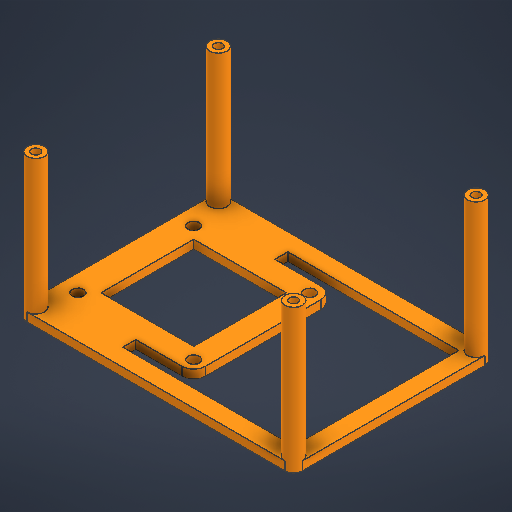
# Autodesk Inventor part: fan_support
Saved by Autodesk Inventor 2026.1 (Build 301233000, 233)
## iProperties
Created: 2026-04-26
Part Number: fan_support
Material: Generic
Document SubType Name: Modeling
Designer: emanuel
Density: 1 g/cm^3
Appearance: Default
Author: emanuel
Autodesk Inventor part; units mm, degrees
ref_plane "YZ Plane" through (0, 0, 0) normal (1, 0, 0) x (0, 1, 0)
ref_plane "XZ Plane" through (0, 0, 0) normal (0, 1, 0) x (-1, 0, 0)
ref_plane "XY Plane" through (0, 0, 0) normal (0, 0, 1) x (1, 0, 0)
sketch "Sketch1" plane through (0, 0, 0) normal (0, 1, 0) x (-1, 0, 0)
  line L0 (0, 0) -> (40, 0)
  line L1 (40, 0) -> (40, -40)
  line L2 (40, -40) -> (0, -40)
  line L3 (0, -40) -> (0, 0)
  circle A0 centre (40, 0) radius 2
  circle A1 centre (40, -40) radius 2
  circle A2 centre (0, -40) radius 2
  circle A3 centre (0, 0) radius 2
  line L4 (40, -20) -> (43, -20)
  line L5 (43, 11.5) -> (43, -51.5)
  circle A4 centre (43, 11.5) radius 1.5
  circle A5 centre (43, -51.5) radius 1.5
  line L6 (43, 11.5) -> (-46, 11.5)
  line L7 (-46, 11.5) -> (-46, -51.5)
  line L8 (-46, -51.5) -> (43, -51.5)
  line L9 (43, -51.5) -> (43, 11.5)
  circle A6 centre (-46, 11.5) radius 1.5
  circle A7 centre (-46, -51.5) radius 1.5
  line L10 (-46, 11.5) -> (-46, -51.5) construction
  line L11 (-49, 11.5) -> (-49, -51.5)
  line L12 (-43, -51.5) -> (-43, 11.5)
  arc A8 (-43, 11.5) -> (-49, 11.5) centre (-46, 11.5) ccw
  arc A9 (-49, -51.5) -> (-43, -51.5) centre (-46, -51.5) ccw
  line L13 (-46, 11.5) -> (43, 11.5) construction
  line L14 (-46, 8.5) -> (43, 8.5)
  line L15 (43, 14.5) -> (-46, 14.5)
  arc A10 (-46, 14.5) -> (-46, 8.5) centre (-46, 11.5) ccw
  arc A11 (43, 8.5) -> (43, 14.5) centre (43, 11.5) ccw
  line L16 (43, 11.5) -> (43, -51.5) construction
  line L17 (40, 11.5) -> (40, -51.5)
  line L18 (46, -51.5) -> (46, 11.5)
  arc A12 (46, 11.5) -> (40, 11.5) centre (43, 11.5) ccw
  arc A13 (40, -51.5) -> (46, -51.5) centre (43, -51.5) ccw
  line L19 (43, -51.5) -> (-46, -51.5) construction
  line L20 (43, -48.5) -> (-46, -48.5)
  line L21 (-46, -54.5) -> (43, -54.5)
  arc A14 (43, -54.5) -> (43, -48.5) centre (43, -51.5) ccw
  arc A15 (-46, -48.5) -> (-46, -54.5) centre (-46, -51.5) ccw
  line L22 (40, 0) -> (0, 0) construction
  line L23 (40, 4) -> (0, 4)
  line L24 (0, -4) -> (40, -4)
  arc A16 (40, -4) -> (40, 4) centre (40, 0) ccw
  arc A17 (0, 4) -> (0, -4) centre (0, 0) ccw
  line L25 (40, 0) -> (40, -40) construction
  line L26 (36, 0) -> (36, -40)
  line L27 (44, -40) -> (44, 0)
  arc A18 (44, 0) -> (36, 0) centre (40, 0) ccw
  arc A19 (36, -40) -> (44, -40) centre (40, -40) ccw
  line L28 (40, -40) -> (0, -40) construction
  line L29 (40, -36) -> (0, -36)
  line L30 (0, -44) -> (40, -44)
  arc A20 (40, -44) -> (40, -36) centre (40, -40) ccw
  arc A21 (0, -36) -> (0, -44) centre (0, -40) ccw
  line L31 (0, -40) -> (0, 0) construction
  line L32 (4, -40) -> (4, 0)
  line L33 (-4, 0) -> (-4, -40)
  arc A22 (-4, -40) -> (4, -40) centre (0, -40) ccw
  arc A23 (4, 0) -> (-4, 0) centre (0, 0) ccw
  line L34 (20, 0) -> (20, 11.5) construction
  line L35 (24, 0) -> (24, 11.5)
  line L36 (16, 11.5) -> (16, 0)
  arc A24 (16, 0) -> (24, 0) centre (20, 0) ccw
  arc A25 (24, 11.5) -> (16, 11.5) centre (20, 11.5) ccw
  line L37 (20, -40) -> (20, -51.5) construction
  line L38 (16, -40) -> (16, -51.5)
  line L39 (24, -51.5) -> (24, -40)
  arc A26 (24, -40) -> (16, -40) centre (20, -40) ccw
  arc A27 (16, -51.5) -> (24, -51.5) centre (20, -51.5) ccw
  line L40 (40, -20) -> (43, -20) construction
  line L41 (40, -24) -> (43, -24)
  line L42 (43, -16) -> (40, -16)
  arc A28 (40, -16) -> (40, -24) centre (40, -20) ccw
  arc A29 (43, -24) -> (43, -16) centre (43, -20) ccw
  point P0 (-46, -20)
  point P1 (-1.5, 11.5)
  point P2 (-1.5, -51.5)
  point P3 (0, -20)
  point P4 (20, 5.75)
  point P5 (20, -45.75)
  point P6 (41.5, -20)
  point P7 (-43, 8.5)
  point P8 (16, 8.5)
  point P9 (16, 4)
  point P10 (16, -44)
  point P11 (16, -48.5)
  point P12 (-43, -48.5)
  point P13 (40, 8.5)
  point P14 (40, -48.5)
  point P15 (24, -48.5)
  point P16 (24, -44)
  point P17 (24, 4)
  point P18 (24, 8.5)
  point P19 (4, -4)
  point P20 (36, -4)
  point P21 (36, -36)
  point P22 (4, -36)
  point P23 (-46, -54.5)
  point P24 (43, -54.5)
  point P25 (22.6458, 14.5)
  point P26 (17.3542, 14.5)
  point P27 (-46, 14.5)
  point P28 (20, -36)
  point P29 (20, -4)
  point P30 (22.6458, -54.5)
  point P31 (17.3542, -54.5)
  point P32 (40, 4)
  point P33 (40, -44)
  point P34 (40, -36)
  point P35 (40, -4)
  point P36 (43, -54.5)
  dimension "d0" = 40
  dimension "d1" = 40
  dimension "d2" = 4
  dimension "d3" = 4
  dimension "d4" = 4
  dimension "d5" = 4
  dimension "d6" = 3
  dimension "d7" = 63
  dimension "d8" = 3
  dimension "d9" = 3
  dimension "d10" = 89
  dimension "d11" = 3
  dimension "d12" = 3
  dimension "d13" = 6
  dimension "d14" = 6
  dimension "d15" = 6
  dimension "d16" = 6
  dimension "d17" = 8
  dimension "d18" = 8
  dimension "d19" = 8
  dimension "d20" = 8
  dimension "d21" = 8
  dimension "d22" = 8
  dimension "d23" = 8
  constraints: 108 end point, 44 point on circle, 44 tangent, 30 centre point, 20 equal length, 13 midpoint, 8 coincident, 7 perpendicular, 3 horizontal, 3 point on line, 1 vertical
  measures "d0" distance of L1.end L2.end
  measures "d1" distance of L0.end L1.end
  measures "d2" diameter of A0
  measures "d3" diameter of A1
  measures "d4" diameter of A2
  measures "d5" diameter of A3
  measures "d6" distance of L4.start L4.end
  measures "d7" distance of L5.start L5.end
  measures "d8" diameter of A4
  measures "d9" diameter of A5
  measures "d10" distance of L8.end L7.end
  measures "d11" diameter of A6
  measures "d12" diameter of A7
  measures "d13" diameter of A9
  measures "d14" diameter of A11
  measures "d15" diameter of A13
  measures "d16" diameter of A15
  measures "d17" diameter of A17
  measures "d18" diameter of A19
  measures "d19" diameter of A21
  measures "d20" diameter of A23
  measures "d21" diameter of A25
  measures "d22" diameter of A27
  measures "d23" diameter of A29
extrude "Extrusion1" add sketch "Sketch1" along normal blind 3 contours A3 L3 A17 A23 L0 | L0 L32 L24 L3 A3 | A23 L23 L36 L0 | L0 A24 L24 L32 | L24 L32 L29 L3 | L3 A21 L33 A17 | L36 L23 L35 L0 | L0 A24 | L29 L32 L2 A2 L3 | L3 A2 L2 A22 A21 | L35 L23 A18 L0 | L0 L26 L24 A24 | L36 L14 L35 L23 | L29 A26 L2 L32 | A18 L17 A0 L0 | L0 A0 L1 L24 L26 | L35 L14 L17 L23 | L36 L6 L35 L14 | L14 L12 L6 L36 | L24 L1 A28 L26 | L29 L26 L2 A26 | A26 L2 | L2 L38 L30 A22 | A16 L5 L1 A0 L17 | L17 L14 L5 A16 | L35 L6 L17 L14 | L14 L7 A6 L6 L12 | L12 L20 L7 L14 | A25 L15 L6 | L6 A8 L15 A25 | A16 L5 L42 L1 | A28 L1 L29 L26 | A28 L1 | L29 L1 A1 L2 L26 | L39 L30 L38 L2 | L2 A19 L30 L39 | L30 L39 L20 L38 | L17 L6 A4 L5 L14 | A16 L5 | L5 A11 L18 A29 L27 A16 | A25 L15 A12 L6 | L20 L38 L8 L12 | L12 L8 A7 L7 L20 | L6 A6 L7 A10 A8 | L7 A15 L11 A10 | L42 L5 L4 L1 | A16 L27 A29 L5 | L41 L5 A20 L1 | L1 L4 L5 L41 | L2 A1 L17 A19 | A20 L5 A19 L17 A1 L1 | L30 L17 L20 L39 | L20 L39 L8 L38 | L5 A4 L6 A12 A11 | A9 A15 L7 A7 L8 | L8 A27 L21 A9 | A29 L27 L5 | A29 L27 A20 L5 | A19 L5 L20 L17 | A20 A19 L5 | L20 L17 L8 L39 | L8 A27 L21 | A29 L18 L27 | A29 L18 A14 L5 A19 L27 | L20 L5 A5 L8 L17 | L8 A13 L21 A27 | L8 A5 L5 A14 A13
sketch "Sketch2" plane through (0, 3, 0) normal (0, 1, 0) x (1, 0, 0)
  circle A0 centre (-43, -11.5) radius 1.5 projected
  arc A1 (-46, -11.5) -> (-43, -14.5) centre (-43, -11.5) ccw projected
  circle A2 centre (-43, -11.5) radius 3
  circle A3 centre (-43, -11.5) radius 1.5
  circle A4 centre (46, -11.5) radius 1.5 projected
  circle A5 centre (46, -11.5) radius 1.5
  circle A6 centre (46, -11.5) radius 3
  circle A7 centre (46, 51.5) radius 1.5 projected
  circle A8 centre (46, 51.5) radius 1.5
  circle A9 centre (46, 51.5) radius 3
  circle A10 centre (-43, 51.5) radius 1.5 projected
  circle A11 centre (-43, 51.5) radius 1.5
  circle A12 centre (-43, 51.5) radius 3
  point P0 (0, 0)
  dimension "d26" = 3
  dimension "d27" = 3
  dimension "d28" = 6
  dimension "d29" = 3
  dimension "d30" = 6
  dimension "d31" = 3
  dimension "d32" = 6
  constraints: 8 coincident, 7 centre point, 3 other
  measures "d26" diameter of A3
  measures "d27" diameter of A5
  measures "d28" diameter of A6
  measures "d29" diameter of A8
  measures "d30" diameter of A9
  measures "d31" diameter of A11
  measures "d32" diameter of A12
extrude "Extrusion2" add sketch "Sketch2" along normal blind 46.5
body "Solid1"
